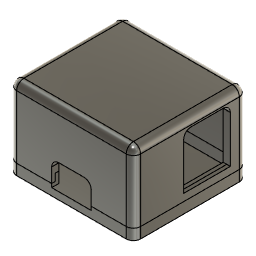
airflow sensor (Autodesk Fusion 360 design; units mm, degrees)
Autodesk Fusion 360 part; units mm, degrees
sketch "Sketch1" plane through (0, 0, 0) normal (0, 0, 1) x (1, 0, 0)
  line L0 (0, 0) -> (34.5, 0)
  line L1 (34.5, 0) -> (34.5, 31.5)
  line L2 (34.5, 31.5) -> (0, 31.5)
  line L3 (0, 31.5) -> (0, 0)
  dimension "d1" = 34.5
  dimension "d2" = 31.5
  constraint horizontal L0
  constraint vertical L1
  constraint horizontal L2
  constraint vertical L3
  constraint coincident L0.start L3.end
  measures "d1" distance of L0.start L0.end
  measures "d2" distance of L0.start L2.end
extrude "Extrude1" add sketch "Sketch1" along normal blind 22.5 makes body 1
shell "Shell1" thickness 2 removed faces 0 bodies 1
ref_plane "WorkPlane1" through (34.5, 15.75, 11.25) normal (1, 0, 0) x (0, 1, 0)
sketch "Sketch2" plane through (34.5, 15.75, 10.5) normal (1, 0, 0) x (0, 1, 0)
  line L0 (-13.75, -8.5) -> (13.75, -8.5)
  line L1 (13.75, -8.5) -> (11.25, -8.5)
  line L2 (13.75, -8.5) -> (-1.75, -8.5)
  line L3 (13.75, -8.5) -> (13.75, -5.5)
  line L4 (13.75, -8.5) -> (13.75, 9.5)
  line L5 (11.25, -5.5) -> (-1.75, -5.5)
  line L6 (-1.75, -5.5) -> (-1.75, 9.5)
  line L7 (-1.75, 9.5) -> (11.25, 9.5)
  line L8 (11.25, 9.5) -> (11.25, -5.5)
  dimension "d7" = 2.5
  dimension "d8" = 15.5
  dimension "d9" = 3
  dimension "d10" = 18
  constraint coincident L0.end L1.start
  constraint parallel L0 L1
  constraint parallel L0 L2
  constraint perpendicular L1 L3
  constraint perpendicular L1 L4
  constraint horizontal L5
  constraint vertical L6
  constraint horizontal L7
  constraint vertical L8
  measures "d7" distance of L0.end L1.end
  measures "d8" distance of L0.end L2.end
  measures "d9" distance of L0.end L3.end
  measures "d10" distance of L0.end L4.end
extrude "Extrude2" cut sketch "Sketch2" against normal blind 49 bodies 1
ref_plane "WorkPlane2" through (17.25, 0, 11.25) normal (0, -1, 0) x (1, 0, 0)
sketch "Sketch3" plane through (17.25, 0, 11.25) normal (0, -1, 0) x (1, 0, 0)
  line L0 (-15.25, -6.25) -> (-17.25, -6.25)
  line L1 (17.25, -6.25) -> (15.25, -6.25)
  line L2 (-15.25, -6.25) -> (15.25, -6.25)
  line L3 (0, -6.25) -> (0, -2.25) construction
  line L4 (0, -6.25) -> (-5.5, -6.25) construction
  line L5 (0, -6.25) -> (5.5, -6.25) construction
  line L6 (-5.5, -2.25) -> (5.5, -2.25)
  line L7 (5.5, -2.25) -> (5.5, -7.2846)
  line L8 (5.5, -7.2846) -> (-5.5, -7.2846)
  line L9 (-5.5, -7.2846) -> (-5.5, -2.25)
  dimension "d14" = 4
  dimension "d15" = 5.5
  dimension "d16" = 5.5
  constraint coincident L0.start L2.start
  constraint coincident L1.end L2.end
  constraint midpoint L2 L3.start
  constraint perpendicular L2 L3
  constraint perpendicular L3 L4
  constraint perpendicular L3 L5
  constraint horizontal L6
  constraint vertical L7
  constraint horizontal L8
  constraint vertical L9
  measures "d14" distance of L3.start L3.end
  measures "d15" distance of L3.start L4.end
  measures "d16" distance of L3.start L5.end
extrude "Extrude3" cut sketch "Sketch3" against normal blind 4.5 contours L2 L6 L7 L9 bodies 1
fillet "Fillet1" radius 2 8 edges at (0, 15.75, 22.5) (34.5, 15.75, 22.5) (17.25, 0, 22.5) (17.25, 31.5, 22.5) (34.5, 0, 11.25) (0, 0, 11.25) (0, 31.5, 11.25) (34.5, 31.5, 11.25) on bodies 1
fillet "Fillet2" radius 2 4 edges at (33.5, 14, 20) (1, 14, 20) (1, 27, 20) (33.5, 27, 20) on bodies 1
ref_plane "WorkPlane3" through (17.25, 15.75, 2) normal (0, 0, 1) x (1, 0, 0)
extrude "Extrude4" cut 1 faces at (15.4167, 0.6667, 5) along direction (0, 0, -1) blind 3 on bodies 1 bodies 1
fillet "Fillet3" radius 2 2 edges at (11.75, 1, 9) (22.75, 1, 9) on bodies 1
split "Split1" by plane through (17.25, 15.75, 2) normal (0, 0, 1) bodies 1 makes body 2 at (12.1667, 11.1667, 22.5)
sketch "Sketch4" plane through (17.25, 15.75, 2) normal (0, 0, 1) x (1, 0, 0)
  line L0 (-15.25, -13.75) -> (-5.5, -13.75)
  line L1 (5.5, -13.75) -> (15.25, -13.75)
  line L2 (15.25, -13.75) -> (15.25, 13.75)
  line L3 (15.25, 13.75) -> (-15.25, 13.75)
  line L4 (-15.25, 13.75) -> (-15.25, -13.75)
  line L5 (5.5, -14.75) -> (16.25, -14.75)
  line L6 (16.25, -14.75) -> (16.25, 14.75)
  line L7 (16.25, 14.75) -> (-16.25, 14.75)
  line L8 (-16.25, 14.75) -> (-16.25, -14.75)
  line L9 (-16.25, -14.75) -> (-5.5, -14.75)
  line L10 (-5.5, -14.75) -> (-5.5, -13.75)
  line L11 (5.5, -14.75) -> (5.5, -13.75)
  dimension "d28" = 1
  constraint coincident L0.end L10.end
  constraint perpendicular L0 L10
  constraint coincident L1.start L11.end
  constraint perpendicular L1 L11
extrude "Extrude5" add sketch "Sketch4" along normal blind 1.5 bodies 1
combine "Combine1" operation cut target body 2 tool bodies 1 keep tools
extrude "Extrude6" add 1 faces at (12.1667, 30.1667, 3.5) along direction (0, 0, 1) blind 1.5 on bodies 1 bodies 1
sketch "Sketch5" plane through (0, 0, 2) normal (0, 0, 1) x (-1, 0, 0)
  line L0 (-33.5, -1) -> (-22.75, -1)
  line L1 (-22.75, -1) -> (-22.75, -2)
  line L2 (-22.75, -2) -> (-32.5, -2)
  line L3 (-32.5, -2) -> (-32.5, -29.5)
  line L4 (-32.5, -29.5) -> (-2, -29.5)
  line L5 (-2, -29.5) -> (-2, -2)
  line L6 (-2, -2) -> (-11.75, -2)
  line L7 (-11.75, -2) -> (-11.75, -1)
  line L8 (-11.75, -1) -> (-1, -1)
  line L9 (-1, -1) -> (-1, -30.5)
  line L10 (-1, -30.5) -> (-33.5, -30.5)
  line L11 (-33.5, -30.5) -> (-33.5, -1)
  line L12 (-2, 0) -> (-32.5, 0)
  arc A0 (-32.5, 0) -> (-34.5, -2) centre (-32.5, -2) ccw
  line L13 (-34.5, -2) -> (-34.5, -29.5)
  arc A1 (-34.5, -29.5) -> (-32.5, -31.5) centre (-32.5, -29.5) ccw
  line L14 (-32.5, -31.5) -> (-2, -31.5)
  arc A2 (-2, -31.5) -> (0, -29.5) centre (-2, -29.5) ccw
  line L15 (0, -29.5) -> (0, -2)
  arc A3 (0, -2) -> (-2, 0) centre (-2, -2) ccw
  line L16 (-11.75, -1) -> (-22.75, -1)
  line L17 (-11.75, -1) -> (-11.75, 0)
  line L18 (-22.75, -1) -> (-22.75, 0)
  constraint coincident L7.end L8.start
  constraint coincident L0.end L1.start
  constraint perpendicular L16 L17
  constraint coincident L12 L18.end
  constraint perpendicular L12 L18
extrude "Extrude7" add sketch "Sketch5" along normal blind 1 contours L0 L8 L9 L10 L11 L12 A0 L13 A1 L14 A2 L15 A3 L17 L18 bodies 1
combine "Combine2" operation cut target body 2 tool bodies 1 keep tools
named bodies: "bot", "top"
